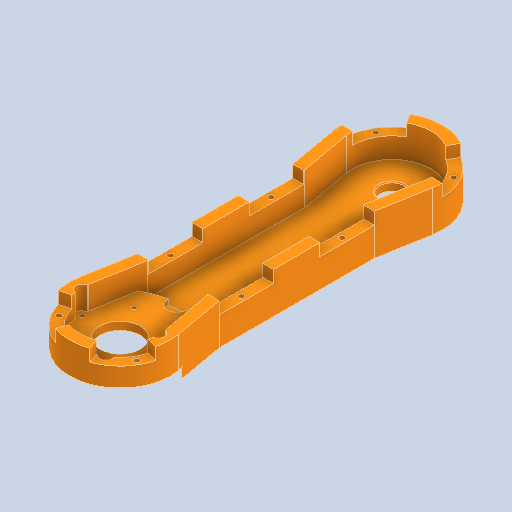
# Autodesk Inventor part: Tercer segmento - superior
Saved by Autodesk Inventor 2026 (Build 300175050, 175E)
## iProperties
Created: 2025-08-11
Part Number: Tercer segmento - superior
Material: Plastico PETG
Document SubType Name: Modeling
Designer: bello
Density: 1.27 g/cm^3
Appearance: Naranja
Author: bello
Autodesk Inventor part; units mm, degrees
ref_plane "YZ Plane" through (0, 0, 0) normal (1, 0, 0) x (0, 1, 0)
ref_plane "XZ Plane" through (0, 0, 0) normal (0, 1, 0) x (-1, 0, 0)
ref_plane "XY Plane" through (0, 0, 0) normal (0, 0, 1) x (1, 0, 0)
sketch "Boceto1" plane through (0, 0, 0) normal (0, 1, 0) x (-1, 0, 0)
  circle A0 centre (0, 0) radius 37
  circle A1 centre (0, -200) radius 37
  line L0 (0, 0) -> (0, -200)
  line L1 (30, -21.6564) -> (30, -178.3436)
  line L2 (-30, -21.6564) -> (-30, -178.3436)
  line L3 (36.4379, -6.425) -> (30, -42.9361)
  line L4 (0, -100) -> (14.5981, -100)
  line L5 (36.4379, -193.575) -> (30, -157.0639)
  line L6 (-36.4379, -6.425) -> (-30, -42.9361)
  line L7 (-36.4379, -193.575) -> (-30, -157.0639)
  point P0 (-36.4379, -6.425)
  point P1 (-30, -42.9361)
  point P2 (-30, -157.0639)
  point P3 (-36.4379, -193.575)
  dimension "d0" = 200
  dimension "d1" = 74
  dimension "d2" = 74
  dimension "d3" = 60
  dimension "d4" = 170
  constraints: 16 end point, 6 symmetric about line, 5 point on circle, 3 parallel, 2 centre point, 1 coincident, 1 horizontal, 1 midpoint, 1 point on line, 1 tangent, 1 vertical
  measures "d0" distance of point (0, 0) L0.end
  measures "d1" diameter of A0
  measures "d2" diameter of A1
  measures "d3" diameter of L1 L0
  measures "d4" angle of L3 L1
extrude "Extrusión1" add sketch "Boceto1" along normal blind 30
sketch "Boceto2" plane through (0, 0, 0) normal (0, -1, 0) x (1, 0, 0)
  circle A0 centre (0, 0) radius 37.1
  dimension "d7" = 74.2
  constraints: 1 centre point, 1 coincident
  measures "d7" diameter of A0
extrude "Extrusión2" cut sketch "Boceto2" against normal blind 7
sketch "Boceto3" plane through (0, 30, 0) normal (0, 1, 0) x (1, 0, 0)
  circle A0 centre (0, 0) radius 43.1
  arc A1 (36.4379, 193.575) -> (-36.4379, 193.575) centre (0, 200) ccw projected
  circle A2 centre (0, 200) radius 29
  line L0 (-28.5594, 194.9642) -> (-22, 157.7639)
  line L1 (-36.4379, 193.575) -> (-30, 157.0639) projected
  line L2 (-22, 157.7639) -> (-22, 42.2361)
  line L3 (-30, 157.0639) -> (-30, 42.9361) projected
  line L4 (0, 0) -> (0, 200)
  line L5 (28.5594, 194.9642) -> (22, 157.7639)
  line L6 (22, 157.7639) -> (22, 42.2361)
  circle A3 centre (0, 0) radius 29
  line L7 (-22, 42.2361) -> (-28.5594, 5.0358)
  line L8 (22, 42.2361) -> (28.5594, 5.0358)
  line L9 (-30, 42.9361) -> (-36.4379, 6.425) projected
  line L10 (36.4379, 6.425) -> (30, 42.9361) projected
  point P0 (-22, 37.0622)
  point P1 (22, 37.0622)
  point P2 (22, 37.0622)
  point P3 (28.5594, 194.9642)
  point P4 (-23.0228, 36.4357)
  point P5 (23.0228, 36.4357)
  dimension "d10" = 86.2
  dimension "d11" = 58
  dimension "d12" = 8
  dimension "d60" = 58
  constraints: 14 end point, 4 parallel, 3 coincident, 3 symmetric about line, 2 point on circle, 2 tangent, 1 centre point, 1 vertical, 7 other
  measures "d12" distance between parallel lines of L2 L3
  measures "d60" diameter of A3
extrude "Extrusión3" cut sketch "Boceto3" against normal blind 24 contours A0 L4 A2 L5 L6 L8 | L7 L2 L0 A2 L4 A0 | A2
sketch "Boceto5" plane through (0, 30, 0) normal (0, 1, 0) x (1, 0, 0)
  circle A0 centre (0, 0) radius 29
  circle A1 centre (0, 0) radius 43.1
  line L0 (-23.0228, 36.4357) -> (-28.5594, 5.0358)
  line L1 (23.0228, 36.4357) -> (28.5594, 5.0358)
  line L2 (-30, 42.9361) -> (-36.4379, 6.425) projected
  line L3 (36.4379, 6.425) -> (30, 42.9361) projected
  dimension "d15" = 58
  dimension "d16" = 86.2
  constraints: 4 end point, 4 point on circle, 2 centre point, 2 coincident, 2 parallel, 2 tangent
  measures "d15" diameter of A0
  measures "d16" diameter of A1
extrude "Extrusión4" cut sketch "Boceto5" against normal blind 17 contours A0 | A0 L0 A1 L1 picked at (2.6828, 38.1473)
sketch "Boceto6" plane through (0, 13, 0) normal (0, 1, 0) x (1, 0, 0)
  circle A0 centre (0, 0) radius 28
  circle A1 centre (14, -24.2487) radius 1.7
  circle A2 centre (28, 0) radius 1.7
  circle A3 centre (14, 24.2487) radius 1.7
  circle A4 centre (-14, 24.2487) radius 1.7
  circle A5 centre (-28, 0) radius 1.7
  circle A6 centre (-14, -24.2487) radius 1.7
  line L0 (-0.7827, -11.2442) -> (-0.7827, 11.3946)
  line L1 (0, 0) -> (-14, -24.2487)
  dimension "d19" = 56
  dimension "d20" = 3.4
  dimension "d23" = 360
  dimension "d34" = 30
  constraints: 6 centre point, 4 end point, 1 coincident, 1 vertical, 16 other
  measures "d20" diameter of A1
  measures "d34" angle of L0 L1
extrude "Extrusión5" cut sketch "Boceto6" along normal through all both and the other way through all contours A0 A2 | A0 A2 | A3 A0 | A0 A3 | A1 A0 | A0 A1 | A4 A0 | A0 A4 | A6 A0 | A0 L1 A6 | A0 A6 L1 | A5 A0 | A0 A5
sketch "Boceto7" plane through (0, 13, 0) normal (0, 1, 0) x (1, 0, 0)
  circle A0 centre (-14, -24.2487) radius 1.7 projected
  circle A1 centre (-14, -24.2487) radius 4.5
  circle A2 centre (14, -24.2487) radius 4.5
  circle A3 centre (28, 0) radius 4.5
  circle A4 centre (14, 24.2487) radius 4.5
  circle A5 centre (-14, 24.2487) radius 4.5
  circle A6 centre (-28, 0) radius 4.5
  point P0 (0, 0)
  dimension "d27" = 9
  dimension "d30" = 360
  constraints: 6 centre point, 1 coincident, 13 other
  measures "d27" diameter of A1
extrude "Extrusión6" cut sketch "Boceto7" along normal through all contours A0 | A1 | A2 | A3 | A4 | A5 | A6
sketch "Boceto8" plane through (0, 13, 0) normal (0, 1, 0) x (1, 0, 0)
  circle A0 centre (0, 0) radius 15
  dimension "d35" = 30
  constraints: 1 centre point, 1 coincident
  measures "d35" diameter of A0
extrude "Extrusión7" cut sketch "Boceto8" against normal through all
sketch "Boceto9" plane through (0, 30, 0) normal (0, 1, 0) x (1, 0, 0)
  arc A0 (28.5594, 194.9642) -> (-28.5594, 194.9642) centre (0, 200) ccw projected
  circle A1 centre (0, 200) radius 29
  circle A2 centre (0, 200) radius 37
  line L0 (0, 200) -> (-18.5, 232.0429)
  line L1 (0, 200) -> (0, 0)
  line L2 (0, 0) -> (-12.6547, -34.7686)
  arc A3 (-36.4379, 6.425) -> (36.4379, 6.425) centre (0, 0) ccw projected
  line L3 (0, 0) -> (-35.7393, -9.5763)
  line L4 (-30, 42.9361) -> (-22, 42.9361)
  line L5 (-22, 42.9361) -> (-22, 82.9361)
  line L6 (-22, 82.9361) -> (-30, 82.9361)
  line L7 (-30, 42.9361) -> (-30, 82.9361)
  line L8 (-30, 157.0639) -> (-22, 157.0639)
  line L9 (-22, 117.0639) -> (-30, 117.0639)
  line L10 (-30, 157.0639) -> (-30, 117.0639)
  line L11 (0, 200) -> (-37, 200)
  line L12 (-22, 117.0639) -> (-22, 157.0639)
  line L13 (-22, 42.2361) -> (-22, 157.7639) projected
  line L14 (0, 200) -> (18.5, 232.0429)
  line L15 (0, 0) -> (12.6547, -34.7686)
  line L16 (0, 0) -> (35.7393, -9.5763)
  line L17 (30, 42.9361) -> (22, 42.9361)
  line L18 (22, 42.9361) -> (22, 82.9361)
  line L19 (22, 82.9361) -> (30, 82.9361)
  line L20 (30, 42.9361) -> (30, 82.9361)
  line L21 (30, 157.0639) -> (22, 157.0639)
  line L22 (22, 117.0639) -> (30, 117.0639)
  line L23 (30, 157.0639) -> (30, 117.0639)
  line L24 (0, 200) -> (37, 200)
  line L25 (22, 117.0639) -> (22, 157.0639)
  circle A4 centre (0, 0) radius 29
  circle A5 centre (0, 0) radius 37
  point P0 (-22, 37.0622)
  point P1 (22, 37.0622)
  point P2 (22, 157.7639)
  point P3 (14.5, 225.1147)
  point P4 (29, 200)
  point P5 (-29, 200)
  point P6 (-14.5, 225.1147)
  point P7 (28.0118, -7.5058)
  point P8 (9.9186, -27.2511)
  point P9 (35.7393, -9.5763)
  point P10 (-9.9186, -27.2511)
  point P11 (-28.0118, -7.5058)
  dimension "d38" = 30
  dimension "d39" = 20
  dimension "d40" = 55
  dimension "d41" = 40
  dimension "d42" = 40
  constraints: 50 end point, 14 symmetric about line, 4 centre point, 4 coincident, 4 point on circle, 3 horizontal, 3 perpendicular, 1 collinear, 1 concentric, 1 parallel, 1 vertical
  measures "d38" angle of L1 L0
  measures "d39" angle of L2 L1
  measures "d40" angle of L2 L3
  measures "d41" distance of L4.end L5.end
  measures "d42" distance of L8.start L9.end
extrude "Extrusión8" cut sketch "Boceto9" against normal blind 9 contours A0 L14 A2 L24 | A0 L11 A2 L0 | A4 L2 A3 L3 | A4 L16 A3 L15 | L7 L6 L5 L4 | L9 L10 L8 L12 | L17 L18 L19 L20 | L23 L22 L25 L21
sketch "Boceto10" plane through (0, 21, 0) normal (0, 1, 0) x (1, 0, 0)
  circle A0 centre (-26, 62.9361) radius 2.05
  circle A1 centre (-26, 137.0639) radius 2.05
  arc A2 (-29, 200) -> (-28.5594, 194.9642) centre (0, 200) ccw projected
  circle A3 centre (0, 200) radius 33
  circle A4 centre (-28.5788, 216.5) radius 2.05
  circle A5 centre (0, 0) radius 33
  circle A6 centre (-28.5788, -16.5) radius 2.05
  line L0 (-30, 42.9361) -> (-30, 82.9361) projected
  line L1 (-30, 82.9361) -> (-22, 82.9361) projected
  line L2 (-30, 117.0639) -> (-30, 157.0639) projected
  line L3 (-22, 117.0639) -> (-30, 117.0639) projected
  line L4 (0, 200) -> (-28.5788, 216.5)
  line L5 (0, 0) -> (-28.5788, -16.5)
  line L6 (0, 0) -> (0, 200)
  circle A7 centre (26, 62.9361) radius 2.05
  circle A8 centre (26, 137.0639) radius 2.05
  circle A9 centre (28.5788, 216.5) radius 2.05
  circle A10 centre (28.5788, -16.5) radius 2.05
  line L7 (0, 200) -> (28.5788, 216.5)
  line L8 (0, 0) -> (28.5788, -16.5)
  dimension "d45" = 66
  dimension "d46" = 66
  dimension "d47" = 4.1
  dimension "d48" = 4
  dimension "d49" = 20
  dimension "d50" = 4
  dimension "d51" = 20
  dimension "d53" = 60
  dimension "d54" = 60
  constraints: 10 end point, 8 centre point, 4 symmetric about line, 3 equal radius, 2 coincident, 1 vertical, 10 other
  measures "d47" diameter of A1
  measures "d48" distance from line of A0.centre L0
  measures "d49" distance from line of L1 A0.centre
  measures "d50" distance from line of L2 A1.centre
  measures "d51" distance from line of L3 A1.centre
  measures "d53" angle of L6 L5
  measures "d54" angle of L6 L4
extrude "Extrusión9" cut sketch "Boceto10" against normal blind 5.8 contours A0 | A1 | A9 L7 A3 | A3 A9 | L7 A9 A3 | A4 A3 | A3 L4 A4 | A3 A4 L4 | A6 L5 A5 | A5 A6 | A10 A5 | A5 L8 A10 | L5 A6 A5 | L8 A5 A10 | A7 | A8
sketch "Boceto11" plane through (0, 6, 0) normal (0, 1, 0) x (1, 0, 0)
  arc A0 (14.5, 225.1147) -> (-14.5, 225.1147) centre (0, 200) ccw projected
  circle A1 centre (0, 200) radius 9
  point P0 (0, 0)
  dimension "d57" = 18
  constraints: 1 centre point, 1 coincident
  measures "d57" diameter of A1
extrude "Extrusión10" cut sketch "Boceto11" against normal through all
sketch "Boceto12" plane through (0, 13, 0) normal (0, 1, 0) x (1, 0, 0)
  circle A0 centre (0, 42) radius 7
  point P0 (0, 0)
  dimension "d61" = 14
  dimension "d62" = 42
  constraints: 1 centre point
  measures "d61" diameter of A0
  measures "d62" distance of point (0, 0) A0.centre
extrude "Extrusión11" cut sketch "Boceto12" against normal blind 4
chamfer "Chaflán1" distance 0.7 angle 45 1 edges at (-9, 6, -200)
equation "\"d5\" = altura"
equation "\"altura\" = 30"
